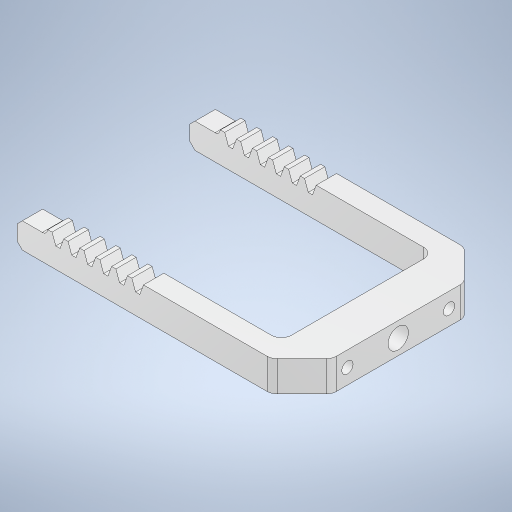
# Autodesk Inventor part: Rack
Saved by Autodesk Inventor 2023.2 (Build 272271000, 271)
## iProperties
Created: 2024-01-11
Part Number: Rack
Material: Aluminum 6061
Document SubType Name: Modeling
Designer: Nathan Cai
Mass: 38.2755 g
Surface Area: 79.1524 cm^2
Volume: 14.1761 cm^3
Density: 2.7 g/cm^3
Appearance: Aluminum - Flat
Author: Nathan Cai
Autodesk Inventor part; units mm, degrees
ref_plane "YZ Plane" through (0, 0, 0) normal (1, 0, 0) x (0, 1, 0)
ref_plane "XZ Plane" through (0, 0, 0) normal (0, 1, 0) x (-1, 0, 0)
ref_plane "XY Plane" through (0, 0, 0) normal (0, 0, 1) x (1, 0, 0)
sketch "Sketch1" plane through (0, 0, 0) normal (0, 1, 0) x (-1, 0, 0)
  line L0 (38.1, 23.8125) -> (-38.1, 23.8125)
  line L1 (-38.1, 23.8125) -> (-38.1, -23.8125)
  line L2 (-38.1, -23.8125) -> (38.1, -23.8125)
  line L3 (38.1, -23.8125) -> (38.1, 23.8125)
  line L4 (38.1, 23.8125) -> (-38.1, -23.8125) construction
  line L5 (-38.1, 23.8125) -> (38.1, -23.8125) construction
  line L6 (0, 0) -> (-38.1, 0) construction
  line L7 (38.1, 30.1625) -> (-50.8, 30.1625)
  line L8 (-50.8, 30.1625) -> (-50.8, -30.1625)
  line L9 (-50.8, -30.1625) -> (38.1, -30.1625)
  line L10 (38.1, -30.1625) -> (38.1, 30.1625)
  line L11 (38.1, 30.1625) -> (-50.8, -30.1625) construction
  line L12 (-50.8, 30.1625) -> (38.1, -30.1625) construction
  point P0 (-6.35, 0)
  point P1 (38.1, 23.8125)
  dimension "d0" = 76.2
  dimension "d1" = 47.625
  dimension "d2" = 6.35
  dimension "d3" = 12.7
  constraints: 26 end point, 5 midpoint, 4 parallel, 2 horizontal, 2 perpendicular, 2 point on line
  measures "d0" distance of L2.end L1.end
  measures "d1" distance of L1.end L0.end
  measures "d2" distance between parallel lines of L2 L9
  measures "d3" distance between parallel lines of L1 L8
extrude "Extrusion1" add sketch "Sketch1" along normal blind 9.525 contours L0 L1 L2 L10 L9 L8 L7
chamfer "Chamfer1" distance 9.525 angle 45 2 edges at (50.8, 4.7625, 30.1625) (50.8, 4.7625, -30.1625)
fillet "Fillet1" radius 3.175 4 edges at (41.275, 4.7625, -30.1625) (50.8, 4.7625, -20.6375) (50.8, 4.7625, 20.6375) (41.275, 4.7625, 30.1625)
fillet "Fillet4" radius 3.175 2 edges at (38.1, 4.7625, -23.8125) (38.1, 4.7625, 23.8125)
sketch "Sketch2" plane through (50.8, 0, 19.3224) normal (1, 0, 0) x (0, 0, -1)
  line L0 (43.1349, 9.525) -> (-4.4901, 9.525) projected
  line L1 (43.1349, 0) -> (-4.4901, 0) projected
  circle A0 centre (19.3224, 4.7625) radius 3.175
  line L2 (0, 9.525) -> (38.6447, 9.525) projected
  line L3 (19.3224, 9.525) -> (19.3224, 0) construction
  line L4 (19.3224, 4.7625) -> (3.4474, 4.7625) construction
  circle A1 centre (3.4474, 4.7625) radius 1.7526
  circle A2 centre (35.1974, 4.7625) radius 1.7526
  point P0 (38.6447, 9.525)
  point P1 (6.35, 9.525)
  point P2 (38.6447, 0)
  point P3 (6.35, 0)
  dimension "d10" = 6.35
  dimension "d99" = 15.875
  dimension "d100" = 3.5052
  dimension "d103" = 360
  constraints: 4 end point, 3 centre point, 3 midpoint, 1 coincident, 1 parallel, 1 perpendicular, 5 other
  measures "d10" diameter of A0
  measures "d99" distance of L4.start L4.end
  measures "d100" diameter of A1
extrude "Extrusion6" cut sketch "Sketch2" against normal through all
sketch "Sketch5" plane through (-38.1, 0, -30.1625) normal (0, 0, -1) x (-1, 0, 0)
  line L0 (0, 0) -> (0, 9.525) projected
  line L1 (0, 9.525) -> (-78.0599, 9.525) projected
  line L2 (-10.8754, 9.525) -> (-12.031, 6.35)
  line L3 (-12.031, 6.35) -> (-13.369, 6.35)
  line L4 (-13.369, 6.35) -> (-14.5246, 9.525)
  line L5 (-25.4, 9.525) -> (-25.4, 6.35) construction
  line L6 (0, 9.525) -> (0, 6.35) construction
  line L7 (-12.7, 9.525) -> (-12.7, 6.35) construction
  line L8 (-25.4, 7.9375) -> (0, 7.9375) construction
  line L9 (-15.8627, 9.525) -> (-17.0183, 6.35)
  line L10 (-17.0183, 6.35) -> (-18.3563, 6.35)
  line L11 (-18.3563, 6.35) -> (-19.5119, 9.525)
  line L12 (-17.6873, 9.525) -> (-17.6873, 6.35) construction
  line L13 (-20.8499, 9.525) -> (-22.0055, 6.35)
  line L14 (-22.0055, 6.35) -> (-23.3436, 6.35)
  line L15 (-23.3436, 6.35) -> (-24.4992, 9.525)
  line L16 (-22.6746, 9.525) -> (-22.6746, 6.35) construction
  line L17 (-25.8372, 9.525) -> (-26.9928, 6.35)
  line L18 (-26.9928, 6.35) -> (-28.3309, 6.35)
  line L19 (-28.3309, 6.35) -> (-29.4865, 9.525)
  line L20 (-27.6618, 9.525) -> (-27.6618, 6.35) construction
  line L21 (-30.8245, 9.525) -> (-31.9801, 6.35)
  line L22 (-31.9801, 6.35) -> (-33.3181, 6.35)
  line L23 (-33.3181, 6.35) -> (-34.4737, 9.525)
  line L24 (-32.6491, 9.525) -> (-32.6491, 6.35) construction
  line L25 (-35.8118, 9.525) -> (-36.9674, 6.35)
  line L26 (-36.9674, 6.35) -> (-38.3054, 6.35)
  line L27 (-38.3054, 6.35) -> (-39.461, 9.525)
  line L28 (-37.6364, 9.525) -> (-37.6364, 6.35) construction
  line L29 (-12.031, 6.35) -> (0, 6.35)
  line L30 (-5.8881, 9.525) -> (-7.0437, 6.35)
  line L31 (-8.3817, 6.35) -> (-9.5373, 9.525)
  line L32 (-8.9595, 7.9375) -> (0, 7.9375)
  point P0 (-38.1, 0)
  point P1 (-13.9468, 7.9375)
  point P2 (-11.4532, 7.9375)
  point P3 (-11.4532, 7.9375)
  point P4 (-16.4405, 7.9375)
  point P5 (-16.4405, 7.9375)
  point P6 (-4.9873, 6.35)
  point P7 (-30.3873, 6.35)
  point P8 (-18.9341, 7.9375)
  point P9 (-21.4277, 7.9375)
  point P10 (-21.4277, 7.9375)
  point P11 (-9.9746, 6.35)
  point P12 (-35.3746, 6.35)
  point P13 (-23.9214, 7.9375)
  point P14 (-26.415, 7.9375)
  point P15 (-26.415, 7.9375)
  point P16 (-14.9618, 6.35)
  point P17 (-40.3618, 6.35)
  point P18 (-28.9087, 7.9375)
  point P19 (-31.4023, 7.9375)
  point P20 (-31.4023, 7.9375)
  point P21 (-19.9491, 6.35)
  point P22 (-45.3491, 6.35)
  point P23 (-33.8959, 7.9375)
  point P24 (-36.3896, 7.9375)
  point P25 (-36.3896, 7.9375)
  point P26 (-24.9364, 6.35)
  point P27 (-50.3364, 6.35)
  point P28 (-38.8832, 7.9375)
  point P29 (-15.8627, 9.525)
  point P30 (-35.8118, 9.525)
  point P31 (-30.8245, 9.525)
  point P32 (-25.8372, 9.525)
  point P33 (-29.4865, 9.525)
  point P34 (-20.8499, 9.525)
  point P35 (-24.4992, 9.525)
  point P36 (-6.4659, 7.9375)
  point P37 (-6.4659, 7.9375)
  point P38 (0, 7.9375)
  point P39 (-9.5373, 9.525)
  dimension "d68" = 3.175
  dimension "d70" = 70
  dimension "d71" = 2.4936
  dimension "d74" = 4.9873
  dimension "d79" = 12.7
  dimension "d82" = 4.9873
  constraints: 62 end point, 19 point on line, 18 midpoint, 4 horizontal, 1 collinear, 1 vertical, 86 other
  measures "d68" distance from line of L1 L6.end
  measures "d70" angle of L3 L2
  measures "d71" distance of point (-11.453, 7.937) point (-13.947, 7.938)
  measures "d74" distance of L2.start L9.start
  measures "d79" distance between parallel lines of L0 L7
  measures "d82" distance of L2.start L30.start
extrude "Extrusion8" cut sketch "Sketch5" against normal through all contours L32 L30 L1 L0 | L32 L31 L1 L30 | L3 L4 L1 L2 | L9 L10 L11 L1 | L13 L14 L15 L1 | L17 L18 L19 L1 | L21 L22 L23 L1 | L25 L26 L27 L1
fillet "Fillet5" radius 1.5875 2 edges at (-29.1405, 7.9375, -26.9875) (-29.1405, 7.9375, 26.9875)
chamfer "Chamfer3" distance 1.5875 angle 45 2 edges at (-38.1, 7.9375, -26.9875) (-38.1, 7.9375, 26.9875)
chamfer "Chamfer4" distance 1.5875 angle 45 2 edges at (-38.1, 0, -26.9875) (-38.1, 0, 26.9875)
ref_plane "Work Plane1" through (39.9599, 0, 14.2875) normal (0, 0, 1) x (1, 0, 0)
sketch "Sketch7" plane through (39.9599, 0, 14.2875) normal (0, 0, 1) x (1, 0, 0)
  line L0 (0, 0) -> (-76.4724, 0) projected
  line L1 (-1.8599, 9.525) -> (-1.8599, 0) projected
  line L2 (-1.8599, 0) -> (2.9026, 0)
  line L3 (2.9026, 0) -> (2.9026, 2.3813) construction
  line L4 (2.9026, 2.3813) -> (-1.8599, 2.3812) construction
  line L5 (-1.8599, 2.3812) -> (-1.8599, 0)
  line L6 (-1.8599, 2.3812) -> (2.9026, 0)
  point P0 (-39.9599, 0)
  point P1 (-1.8599, 2.3812)
  dimension "d114" = 4.7625
  dimension "d115" = 2.3813
  constraints: 10 end point, 2 parallel, 1 horizontal, 1 perpendicular
  measures "d114" distance of L4.end L3.end
  measures "d115" distance of L3.end L2.end
extrude "Extrusion10" cut sketch "Sketch7" against normal blind 9.525
mirror "Mirror2" about plane through (0, 0, 0) normal (0, 0, 1) of "Extrusion10"
equation "\"d71\" = 0.5 * d69"
equation "\"d74\" = 1.5708 * d68"
equation "\"d82\" = d74"
equation "\"d69\" = 1.5708 * d68"
body "Solid1"
